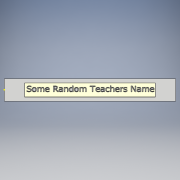
# Autodesk Inventor part: NameTag
Saved by Autodesk Inventor 2018 (Build 220112000, 112)
## iProperties
Created: 2019-03-18
Part Number: NameTag
Material: Generic
Document SubType Name: Modeling
Designer: This kid
Density: 1 g/cm^3
Appearance: Default
Author: This kid
Autodesk Inventor part; units mm, degrees
(part 1 of 2)
ref_plane "YZ Plane" through (0, 0, 0) normal (1, 0, 0) x (0, 1, 0)
ref_plane "XZ Plane" through (0, 0, 0) normal (0, 1, 0) x (-1, 0, 0)
ref_plane "XY Plane" through (0, 0, 0) normal (0, 0, 1) x (1, 0, 0)
sketch "Sketch1" plane through (0, 0, 0) normal (0, 0, 1) x (1, 0, 0)
  line L0 (0, 6.6514) -> (5.7603, -3.3257)
  line L1 (5.7603, -3.3257) -> (-5.7603, -3.3257)
  line L2 (-5.7603, -3.3257) -> (0, 6.6514)
  point P0 (0, 0)
  point P1 (0, 0)
  constraints: 6 end point, 1 coincident, 7 other
extrude "Extrusion1" add sketch "Sketch1" along normal blind 76.2
sketch "Sketch2" plane through (-5.7603, -3.3257, 0) normal (-0.8660254, 0.5, 0) x (0, 0, 1)
  line L0 (9.0292, 2.0917) -> (67.1704, 2.0917)
  line L1 (67.1704, 2.0917) -> (67.1704, 9.2481)
  line L2 (67.1704, 9.2481) -> (9.0292, 9.2481)
  line L3 (9.0292, 9.2481) -> (9.0292, 2.0917)
  line L4 (0, 5.7603) -> (9.0292, 5.6699) construction
  line L5 (67.1704, 5.7603) -> (76.2, 5.7603) construction
  constraints: 12 end point, 2 parallel, 1 equal length, 1 horizontal, 1 midpoint, 1 perpendicular, 1 point on line
extrude "Extrusion2" add sketch "Sketch2" along normal blind 0.2286
sketch "Sketch3" plane through (-5.9582, -3.2114, 0) normal (-0.8660254, 0.5, 0) x (0, 0, 1)
  point P0 (0, 5.7603)
sketch "Sketch4" plane through (-5.9582, -3.2114, 0) normal (-0.8660254, 0.5, 0) x (0, 0, 1)
  line L0 (9.8332, 7.8709) -> (68.5929, 7.8709) construction
  line L1 (68.5929, 7.8709) -> (68.5929, 1.5104) construction
  line L2 (68.5929, 1.5104) -> (9.8332, 1.5104) construction
  line L3 (9.8332, 1.5104) -> (9.8332, 7.8709) construction
  spline S0 degree 2 poles (10.9916, 4.6327) (10.6607, 4.6327) (10.1963, 4.7711) (9.9913, 4.8699) knots 0 0 0 1 2 2 2
  line L4 (9.9913, 4.8699) -> (9.9913, 5.3787)
  line L5 (9.9913, 5.3787) -> (10.0209, 5.3787)
  spline S1 degree 2 poles (10.0209, 5.3787) (10.221, 5.191) (10.7274, 4.9835) (10.962, 4.9835) knots 0 0 0 1 2 2 2
  spline S2 degree 2 poles (10.962, 4.9835) (11.2979, 4.9835) (11.6413, 5.2626) (11.6413, 5.4923) knots 0 0 0 1 2 2 2
  spline S3 degree 2 poles (11.6413, 5.4923) (11.6413, 5.6751) (11.4609, 5.9023) (11.2658, 5.9591) knots 0 0 0 1 2 2 2
  spline S4 degree 2 poles (11.2658, 5.9591) (11.125, 5.9987) (10.8904, 6.053) (10.715, 6.0975) knots 0 0 0 1 2 2 2
  spline S5 degree 2 poles (10.715, 6.0975) (10.5569, 6.1394) (10.3075, 6.2654) (10.2111, 6.3667) knots 0 0 0 1 2 2 2
  spline S6 degree 2 poles (10.2111, 6.3667) (10.1173, 6.468) (10.0135, 6.7397) (10.0135, 6.9175) knots 0 0 0 1 2 2 2
  spline S7 degree 2 poles (10.0135, 6.9175) (10.0135, 7.288) (10.5915, 7.7894) (11.0386, 7.7894) knots 0 0 0 1 2 2 2
  spline S8 degree 2 poles (11.0386, 7.7894) (11.2955, 7.7894) (11.7499, 7.6881) (11.9451, 7.5918) knots 0 0 0 1 2 2 2
  line L6 (11.9451, 7.5918) -> (11.9451, 7.1077)
  line L7 (11.9451, 7.1077) -> (11.9154, 7.1077)
  spline S9 degree 2 poles (11.9154, 7.1077) (11.7697, 7.2411) (11.3152, 7.4387) (11.0657, 7.4387) knots 0 0 0 1 2 2 2
  spline S10 degree 2 poles (11.0657, 7.4387) (10.7842, 7.4387) (10.4359, 7.1744) (10.4359, 6.9595) knots 0 0 0 1 2 2 2
  spline S11 degree 2 poles (10.4359, 6.9595) (10.4359, 6.7668) (10.6409, 6.5371) (10.8336, 6.4852) knots 0 0 0 1 2 2 2
  spline S12 degree 2 poles (10.8336, 6.4852) (10.962, 6.4507) (11.335, 6.3617) (11.4585, 6.3247) knots 0 0 0 1 2 2 2
  spline S13 degree 2 poles (11.4585, 6.3247) (11.7722, 6.2284) (12.0636, 5.8406) (12.0636, 5.5565) knots 0 0 0 1 2 2 2
  spline S14 degree 2 poles (12.0636, 5.5565) (12.0636, 5.3762) (11.9179, 5.0304) (11.787, 4.9094) knots 0 0 0 1 2 2 2
  spline S15 degree 2 poles (11.787, 4.9094) (11.6413, 4.776) (11.2708, 4.6327) (10.9916, 4.6327) knots 0 0 0 1 2 2 2
  spline S16 degree 2 poles (14.3262, 5.8307) (14.3262, 5.2527) (13.7704, 4.6229) (13.3061, 4.6229) knots 0 0 0 1 2 2 2
  spline S17 degree 2 poles (13.3061, 4.6229) (12.8293, 4.6229) (12.2835, 5.2725) (12.2835, 5.8307) knots 0 0 0 1 2 2 2
  spline S18 degree 2 poles (12.2835, 5.8307) (12.2835, 6.4037) (12.8466, 7.0385) (13.3061, 7.0385) knots 0 0 0 1 2 2 2
  spline S19 degree 2 poles (13.3061, 7.0385) (13.7704, 7.0385) (14.3262, 6.4062) (14.3262, 5.8307) knots 0 0 0 1 2 2 2
  spline S20 degree 2 poles (13.9285, 5.8307) (13.9285, 6.2753) (13.6049, 6.7075) (13.3061, 6.7075) knots 0 0 0 1 2 2 2
  spline S21 degree 2 poles (13.3061, 6.7075) (13.0072, 6.7075) (12.6811, 6.2753) (12.6811, 5.8307) knots 0 0 0 1 2 2 2
  spline S22 degree 2 poles (12.6811, 5.8307) (12.6811, 5.3984) (13.0072, 4.9538) (13.3061, 4.9538) knots 0 0 0 1 2 2 2
  spline S23 degree 2 poles (13.3061, 4.9538) (13.6025, 4.9538) (13.9285, 5.391) (13.9285, 5.8307) knots 0 0 0 1 2 2 2
  line L8 (17.3149, 4.6871) -> (17.3149, 6.011)
  spline S24 degree 2 poles (17.3149, 6.011) (17.3149, 6.1691) (17.2902, 6.4383) (17.2507, 6.5124) knots 0 0 0 1 2 2 2
  spline S25 degree 2 poles (17.2507, 6.5124) (17.2111, 6.5939) (17.0605, 6.673) (16.9296, 6.673) knots 0 0 0 1 2 2 2
  spline S26 degree 2 poles (16.9296, 6.673) (16.811, 6.673) (16.5393, 6.5272) (16.396, 6.3889) knots 0 0 0 1 2 2 2
  spline S27 degree 2 poles (16.396, 6.3889) (16.3985, 6.3543) (16.4035, 6.258) (16.4035, 6.1938) knots 0 0 0 1 2 2 2
  line L9 (16.4035, 6.1938) -> (16.4035, 4.6871)
  line L10 (16.4035, 4.6871) -> (16.0181, 4.6871)
  line L11 (16.0181, 4.6871) -> (16.0181, 6.011)
  spline S28 degree 2 poles (16.0181, 6.011) (16.0181, 6.1691) (15.9934, 6.4383) (15.9539, 6.5124) knots 0 0 0 1 2 2 2
  spline S29 degree 2 poles (15.9539, 6.5124) (15.9144, 6.5939) (15.7637, 6.673) (15.6328, 6.673) knots 0 0 0 1 2 2 2
  spline S30 degree 2 poles (15.6328, 6.673) (15.5093, 6.673) (15.2351, 6.5174) (15.1067, 6.3963) knots 0 0 0 1 2 2 2
  line L12 (15.1067, 6.3963) -> (15.1067, 4.6871)
  line L13 (15.1067, 4.6871) -> (14.7214, 4.6871)
  line L14 (14.7214, 4.6871) -> (14.7214, 6.9743)
  line L15 (14.7214, 6.9743) -> (15.1067, 6.9743)
  line L16 (15.1067, 6.9743) -> (15.1067, 6.7224)
  spline S31 degree 2 poles (15.1067, 6.7224) (15.2574, 6.873) (15.5538, 7.0385) (15.7316, 7.0385) knots 0 0 0 1 2 2 2
  spline S32 degree 2 poles (15.7316, 7.0385) (15.9341, 7.0385) (16.2478, 6.8533) (16.3294, 6.6433) knots 0 0 0 1 2 2 2
  spline S33 degree 2 poles (16.3294, 6.6433) (16.5047, 6.8385) (16.8357, 7.0385) (17.0284, 7.0385) knots 0 0 0 1 2 2 2
  spline S34 degree 2 poles (17.0284, 7.0385) (17.1766, 7.0385) (17.4186, 6.9471) (17.5075, 6.8434) knots 0 0 0 1 2 2 2
  spline S35 degree 2 poles (17.5075, 6.8434) (17.5989, 6.7397) (17.7002, 6.4284) (17.7002, 6.1938) knots 0 0 0 1 2 2 2
  line L17 (17.7002, 6.1938) -> (17.7002, 4.6871)
  line L18 (17.7002, 4.6871) -> (17.3149, 4.6871)
  spline S36 degree 2 poles (19.2341, 4.6352) (18.6857, 4.6352) (18.0831, 5.2502) (18.0831, 5.8183) knots 0 0 0 1 2 2 2
  spline S37 degree 2 poles (18.0831, 5.8183) (18.0831, 6.3766) (18.6685, 7.0385) (19.1402, 7.0385) knots 0 0 0 1 2 2 2
  spline S38 degree 2 poles (19.1402, 7.0385) (19.3527, 7.0385) (19.6812, 6.915) (19.8022, 6.7841) knots 0 0 0 1 2 2 2
  spline S39 degree 2 poles (19.8022, 6.7841) (19.9257, 6.6532) (20.0566, 6.2753) (20.0566, 6.0011) knots 0 0 0 1 2 2 2
  line L19 (20.0566, 6.0011) -> (20.0566, 5.7912)
  line L20 (20.0566, 5.7912) -> (18.4733, 5.7912)
  spline S40 degree 2 poles (18.4733, 5.7912) (18.4733, 5.3935) (18.8735, 4.9711) (19.2292, 4.9711) knots 0 0 0 1 2 2 2
  spline S41 degree 2 poles (19.2292, 4.9711) (19.3551, 4.9711) (19.5997, 5.0279) (19.6985, 5.0724) knots 0 0 0 1 2 2 2
  spline S42 degree 2 poles (19.6985, 5.0724) (19.8022, 5.1218) (19.9455, 5.2082) (19.9924, 5.2478) knots 0 0 0 1 2 2 2
  line L21 (19.9924, 5.2478) -> (20.0146, 5.2478)
  line L22 (20.0146, 5.2478) -> (20.0146, 4.8279)
  spline S43 degree 2 poles (20.0146, 4.8279) (19.9479, 4.8007) (19.7454, 4.7217) (19.6663, 4.6994) knots 0 0 0 1 2 2 2
  spline S44 degree 2 poles (19.6663, 4.6994) (19.5552, 4.6673) (19.3724, 4.6352) (19.2341, 4.6352) knots 0 0 0 1 2 2 2
  spline S45 degree 2 poles (19.6812, 6.0851) (19.6762, 6.2407) (19.612, 6.468) (19.5503, 6.5445) knots 0 0 0 1 2 2 2
  spline S46 degree 2 poles (19.5503, 6.5445) (19.4836, 6.631) (19.2736, 6.7224) (19.118, 6.7224) knots 0 0 0 1 2 2 2
  spline S47 degree 2 poles (19.118, 6.7224) (18.9649, 6.7224) (18.75, 6.631) (18.661, 6.5421) knots 0 0 0 1 2 2 2
  spline S48 degree 2 poles (18.661, 6.5421) (18.5746, 6.4507) (18.4857, 6.2308) (18.4733, 6.0851) knots 0 0 0 1 2 2 2
  line L23 (18.4733, 6.0851) -> (19.6812, 6.0851)
  line L24 (24.1445, 4.6871) -> (23.6184, 4.6871)
  line L25 (23.6184, 4.6871) -> (22.6551, 5.8999)
  line L26 (22.6551, 5.8999) -> (22.1907, 5.8999)
  line L27 (22.1907, 5.8999) -> (22.1907, 4.6871)
  line L28 (22.1907, 4.6871) -> (21.7856, 4.6871)
  line L29 (21.7856, 4.6871) -> (21.7856, 7.7351)
  line L30 (21.7856, 7.7351) -> (22.5711, 7.7351)
  spline S49 degree 2 poles (22.5711, 7.7351) (22.8329, 7.7351) (23.1861, 7.6783) (23.3467, 7.5745) knots 0 0 0 1 2 2 2
  spline S50 degree 2 poles (23.3467, 7.5745) (23.5072, 7.4708) (23.6925, 7.1472) (23.6925, 6.9076) knots 0 0 0 1 2 2 2
  spline S51 degree 2 poles (23.6925, 6.9076) (23.6925, 6.5742) (23.3516, 6.1222) (23.0601, 6.0135) knots 0 0 0 1 2 2 2
  line L31 (23.0601, 6.0135) -> (24.1445, 4.6871)
  spline S52 degree 2 poles (23.2701, 6.8755) (23.2701, 7.0089) (23.1762, 7.2139) (23.0774, 7.2806) knots 0 0 0 1 2 2 2
  spline S53 degree 2 poles (23.0774, 7.2806) (22.991, 7.3374) (22.7613, 7.3843) (22.5933, 7.3843) knots 0 0 0 1 2 2 2
  line L32 (22.5933, 7.3843) -> (22.1907, 7.3843)
  line L33 (22.1907, 7.3843) -> (22.1907, 6.2382)
  line L34 (22.1907, 6.2382) -> (22.5464, 6.2382)
  spline S54 degree 2 poles (22.5464, 6.2382) (22.7218, 6.2382) (23.0009, 6.3) (23.0972, 6.3963) knots 0 0 0 1 2 2 2
  spline S55 degree 2 poles (23.0972, 6.3963) (23.1861, 6.4803) (23.2701, 6.7174) (23.2701, 6.8755) knots 0 0 0 1 2 2 2
  spline S56 degree 2 poles (25.6314, 4.9291) (25.5845, 4.8946) (25.4264, 4.7711) (25.3523, 4.734) knots 0 0 0 1 2 2 2
  spline S57 degree 2 poles (25.3523, 4.734) (25.2511, 4.6797) (25.0609, 4.6229) (24.888, 4.6229) knots 0 0 0 1 2 2 2
  spline S58 degree 2 poles (24.888, 4.6229) (24.7472, 4.6229) (24.4928, 4.7291) (24.3964, 4.8254) knots 0 0 0 1 2 2 2
  spline S59 degree 2 poles (24.3964, 4.8254) (24.305, 4.9193) (24.1939, 5.1959) (24.1939, 5.349) knots 0 0 0 1 2 2 2
  spline S60 degree 2 poles (24.1939, 5.349) (24.1939, 5.5862) (24.394, 5.9221) (24.6113, 6.0184) knots 0 0 0 1 2 2 2
  spline S61 degree 2 poles (24.6113, 6.0184) (24.804, 6.1073) (25.3276, 6.174) (25.6314, 6.1913) knots 0 0 0 1 2 2 2
  line L35 (25.6314, 6.1913) -> (25.6314, 6.2654)
  spline S62 degree 2 poles (25.6314, 6.2654) (25.6314, 6.3988) (25.5499, 6.5643) (25.4758, 6.6112) knots 0 0 0 1 2 2 2
  spline S63 degree 2 poles (25.4758, 6.6112) (25.4017, 6.6581) (25.1893, 6.6878) (25.0757, 6.6878) knots 0 0 0 1 2 2 2
  spline S64 degree 2 poles (25.0757, 6.6878) (24.9423, 6.6878) (24.5817, 6.6087) (24.4014, 6.5322) knots 0 0 0 1 2 2 2
  line L36 (24.4014, 6.5322) -> (24.3791, 6.5322)
  line L37 (24.3791, 6.5322) -> (24.3791, 6.9249)
  spline S65 degree 2 poles (24.3791, 6.9249) (24.4853, 6.9546) (24.883, 7.0287) (25.0781, 7.0287) knots 0 0 0 1 2 2 2
  spline S66 degree 2 poles (25.0781, 7.0287) (25.3153, 7.0287) (25.6388, 6.9546) (25.7673, 6.8582) knots 0 0 0 1 2 2 2
  spline S67 degree 2 poles (25.7673, 6.8582) (25.8933, 6.7644) (26.0168, 6.4655) (26.0168, 6.2506) knots 0 0 0 1 2 2 2
  line L38 (26.0168, 6.2506) -> (26.0168, 4.6871)
  line L39 (26.0168, 4.6871) -> (25.6314, 4.6871)
  line L40 (25.6314, 4.6871) -> (25.6314, 4.9291)
  line L41 (25.6314, 5.2502) -> (25.6314, 5.885)
  spline S68 degree 2 poles (25.6314, 5.885) (25.4931, 5.8727) (25.0757, 5.8307) (24.9448, 5.7912) knots 0 0 0 1 2 2 2
  spline S69 degree 2 poles (24.9448, 5.7912) (24.7916, 5.7442) (24.5916, 5.5491) (24.5916, 5.3762) knots 0 0 0 1 2 2 2
  spline S70 degree 2 poles (24.5916, 5.3762) (24.5916, 5.1786) (24.8139, 4.9785) (25.0263, 4.9785) knots 0 0 0 1 2 2 2
  spline S71 degree 2 poles (25.0263, 4.9785) (25.2066, 4.9785) (25.503, 5.1341) (25.6314, 5.2502) knots 0 0 0 1 2 2 2
  line L42 (28.3534, 4.6871) -> (27.9681, 4.6871)
  line L43 (27.9681, 4.6871) -> (27.9681, 5.9912)
  spline S72 degree 2 poles (27.9681, 5.9912) (27.9681, 6.1493) (27.9384, 6.421) (27.894, 6.5025) knots 0 0 0 1 2 2 2
  spline S73 degree 2 poles (27.894, 6.5025) (27.847, 6.589) (27.6791, 6.673) (27.5358, 6.673) knots 0 0 0 1 2 2 2
  spline S74 degree 2 poles (27.5358, 6.673) (27.3926, 6.673) (27.0887, 6.5198) (26.943, 6.3963) knots 0 0 0 1 2 2 2
  line L44 (26.943, 6.3963) -> (26.943, 4.6871)
  line L45 (26.943, 4.6871) -> (26.5577, 4.6871)
  line L46 (26.5577, 4.6871) -> (26.5577, 6.9743)
  line L47 (26.5577, 6.9743) -> (26.943, 6.9743)
  line L48 (26.943, 6.9743) -> (26.943, 6.7199)
  spline S75 degree 2 poles (26.943, 6.7199) (27.1159, 6.8755) (27.4494, 7.0385) (27.6371, 7.0385) knots 0 0 0 1 2 2 2
  spline S76 degree 2 poles (27.6371, 7.0385) (27.973, 7.0385) (28.3534, 6.5939) (28.3534, 6.1716) knots 0 0 0 1 2 2 2
  line L49 (28.3534, 6.1716) -> (28.3534, 4.6871)
  line L50 (30.653, 4.6871) -> (30.2677, 4.6871)
  line L51 (30.2677, 4.6871) -> (30.2677, 4.9193)
  spline S77 degree 2 poles (30.2677, 4.9193) (30.1787, 4.8452) (30.0478, 4.7464) (29.9589, 4.7044) knots 0 0 0 1 2 2 2
  spline S78 degree 2 poles (29.9589, 4.7044) (29.8774, 4.6648) (29.702, 4.6229) (29.5859, 4.6229) knots 0 0 0 1 2 2 2
  spline S79 degree 2 poles (29.5859, 4.6229) (29.3982, 4.6229) (29.082, 4.7785) (28.9709, 4.9291) knots 0 0 0 1 2 2 2
  spline S80 degree 2 poles (28.9709, 4.9291) (28.8597, 5.0798) (28.7362, 5.5244) (28.7362, 5.8134) knots 0 0 0 1 2 2 2
  spline S81 degree 2 poles (28.7362, 5.8134) (28.7362, 6.1147) (28.8919, 6.5544) (29.0277, 6.7199) knots 0 0 0 1 2 2 2
  spline S82 degree 2 poles (29.0277, 6.7199) (29.1537, 6.8681) (29.5069, 7.0385) (29.702, 7.0385) knots 0 0 0 1 2 2 2
  spline S83 degree 2 poles (29.702, 7.0385) (29.8725, 7.0385) (30.1269, 6.962) (30.2677, 6.8829) knots 0 0 0 1 2 2 2
  line L52 (30.2677, 6.8829) -> (30.2677, 7.8709)
  line L53 (30.2677, 7.8709) -> (30.653, 7.8709)
  line L54 (30.653, 7.8709) -> (30.653, 4.6871)
  line L55 (30.2677, 5.2428) -> (30.2677, 6.5643)
  spline S84 degree 2 poles (30.2677, 6.5643) (30.1244, 6.6334) (29.8972, 6.6853) (29.7662, 6.6853) knots 0 0 0 1 2 2 2
  spline S85 degree 2 poles (29.7662, 6.6853) (29.4698, 6.6853) (29.1339, 6.2407) (29.1339, 5.8208) knots 0 0 0 1 2 2 2
  spline S86 degree 2 poles (29.1339, 5.8208) (29.1339, 5.4157) (29.3908, 4.9884) (29.6748, 4.9884) knots 0 0 0 1 2 2 2
  spline S87 degree 2 poles (29.6748, 4.9884) (29.8255, 4.9884) (30.1318, 5.1267) (30.2677, 5.2428) knots 0 0 0 1 2 2 2
  spline S88 degree 2 poles (33.0909, 5.8307) (33.0909, 5.2527) (32.5351, 4.6229) (32.0708, 4.6229) knots 0 0 0 1 2 2 2
  spline S89 degree 2 poles (32.0708, 4.6229) (31.5941, 4.6229) (31.0482, 5.2725) (31.0482, 5.8307) knots 0 0 0 1 2 2 2
  spline S90 degree 2 poles (31.0482, 5.8307) (31.0482, 6.4037) (31.6113, 7.0385) (32.0708, 7.0385) knots 0 0 0 1 2 2 2
  spline S91 degree 2 poles (32.0708, 7.0385) (32.5351, 7.0385) (33.0909, 6.4062) (33.0909, 5.8307) knots 0 0 0 1 2 2 2
  spline S92 degree 2 poles (32.6932, 5.8307) (32.6932, 6.2753) (32.3696, 6.7075) (32.0708, 6.7075) knots 0 0 0 1 2 2 2
  spline S93 degree 2 poles (32.0708, 6.7075) (31.7719, 6.7075) (31.4459, 6.2753) (31.4459, 5.8307) knots 0 0 0 1 2 2 2
  spline S94 degree 2 poles (31.4459, 5.8307) (31.4459, 5.3984) (31.7719, 4.9538) (32.0708, 4.9538) knots 0 0 0 1 2 2 2
  spline S95 degree 2 poles (32.0708, 4.9538) (32.3672, 4.9538) (32.6932, 5.391) (32.6932, 5.8307) knots 0 0 0 1 2 2 2
  line L56 (36.0796, 4.6871) -> (36.0796, 6.011)
  spline S96 degree 2 poles (36.0796, 6.011) (36.0796, 6.1691) (36.0549, 6.4383) (36.0154, 6.5124) knots 0 0 0 1 2 2 2
  spline S97 degree 2 poles (36.0154, 6.5124) (35.9759, 6.5939) (35.8252, 6.673) (35.6943, 6.673) knots 0 0 0 1 2 2 2
  spline S98 degree 2 poles (35.6943, 6.673) (35.5757, 6.673) (35.304, 6.5272) (35.1608, 6.3889) knots 0 0 0 1 2 2 2
  spline S99 degree 2 poles (35.1608, 6.3889) (35.1632, 6.3543) (35.1682, 6.258) (35.1682, 6.1938) knots 0 0 0 1 2 2 2
  line L57 (35.1682, 6.1938) -> (35.1682, 4.6871)
  line L58 (35.1682, 4.6871) -> (34.7828, 4.6871)
  line L59 (34.7828, 4.6871) -> (34.7828, 6.011)
  spline S100 degree 2 poles (34.7828, 6.011) (34.7828, 6.1691) (34.7581, 6.4383) (34.7186, 6.5124) knots 0 0 0 1 2 2 2
  spline S101 degree 2 poles (34.7186, 6.5124) (34.6791, 6.5939) (34.5284, 6.673) (34.3975, 6.673) knots 0 0 0 1 2 2 2
  spline S102 degree 2 poles (34.3975, 6.673) (34.274, 6.673) (33.9998, 6.5174) (33.8714, 6.3963) knots 0 0 0 1 2 2 2
  line L60 (33.8714, 6.3963) -> (33.8714, 4.6871)
  line L61 (33.8714, 4.6871) -> (33.4861, 4.6871)
  line L62 (33.4861, 4.6871) -> (33.4861, 6.9743)
  line L63 (33.4861, 6.9743) -> (33.8714, 6.9743)
  line L64 (33.8714, 6.9743) -> (33.8714, 6.7224)
  spline S103 degree 2 poles (33.8714, 6.7224) (34.0221, 6.873) (34.3185, 7.0385) (34.4963, 7.0385) knots 0 0 0 1 2 2 2
  spline S104 degree 2 poles (34.4963, 7.0385) (34.6989, 7.0385) (35.0126, 6.8533) (35.0941, 6.6433) knots 0 0 0 1 2 2 2
  spline S105 degree 2 poles (35.0941, 6.6433) (35.2694, 6.8385) (35.6004, 7.0385) (35.7931, 7.0385) knots 0 0 0 1 2 2 2
  spline S106 degree 2 poles (35.7931, 7.0385) (35.9413, 7.0385) (36.1833, 6.9471) (36.2723, 6.8434) knots 0 0 0 1 2 2 2
  spline S107 degree 2 poles (36.2723, 6.8434) (36.3637, 6.7397) (36.4649, 6.4284) (36.4649, 6.1938) knots 0 0 0 1 2 2 2
  line L65 (36.4649, 6.1938) -> (36.4649, 4.6871)
  line L66 (36.4649, 4.6871) -> (36.0796, 4.6871)
  line L67 (39.056, 4.6871) -> (39.056, 7.3745)
  line L68 (39.056, 7.3745) -> (38.0334, 7.3745)
  line L69 (38.0334, 7.3745) -> (38.0334, 7.7351)
  line L70 (38.0334, 7.7351) -> (40.4836, 7.7351)
  line L71 (40.4836, 7.7351) -> (40.4836, 7.3745)
  line L72 (40.4836, 7.3745) -> (39.4611, 7.3745)
  line L73 (39.4611, 7.3745) -> (39.4611, 4.6871)
  line L74 (39.4611, 4.6871) -> (39.056, 4.6871)
  spline S108 degree 2 poles (41.7557, 4.6352) (41.2074, 4.6352) (40.6047, 5.2502) (40.6047, 5.8183) knots 0 0 0 1 2 2 2
  spline S109 degree 2 poles (40.6047, 5.8183) (40.6047, 6.3766) (41.1901, 7.0385) (41.6618, 7.0385) knots 0 0 0 1 2 2 2
  spline S110 degree 2 poles (41.6618, 7.0385) (41.8743, 7.0385) (42.2028, 6.915) (42.3238, 6.7841) knots 0 0 0 1 2 2 2
  spline S111 degree 2 poles (42.3238, 6.7841) (42.4473, 6.6532) (42.5782, 6.2753) (42.5782, 6.0011) knots 0 0 0 1 2 2 2
  line L75 (42.5782, 6.0011) -> (42.5782, 5.7912)
  line L76 (42.5782, 5.7912) -> (40.9949, 5.7912)
  spline S112 degree 2 poles (40.9949, 5.7912) (40.9949, 5.3935) (41.3951, 4.9711) (41.7508, 4.9711) knots 0 0 0 1 2 2 2
  spline S113 degree 2 poles (41.7508, 4.9711) (41.8767, 4.9711) (42.1213, 5.0279) (42.2201, 5.0724) knots 0 0 0 1 2 2 2
  spline S114 degree 2 poles (42.2201, 5.0724) (42.3238, 5.1218) (42.4671, 5.2082) (42.514, 5.2478) knots 0 0 0 1 2 2 2
  line L77 (42.514, 5.2478) -> (42.5362, 5.2478)
  line L78 (42.5362, 5.2478) -> (42.5362, 4.8279)
  spline S115 degree 2 poles (42.5362, 4.8279) (42.4695, 4.8007) (42.267, 4.7217) (42.188, 4.6994) knots 0 0 0 1 2 2 2
  spline S116 degree 2 poles (42.188, 4.6994) (42.0768, 4.6673) (41.894, 4.6352) (41.7557, 4.6352) knots 0 0 0 1 2 2 2
  spline S117 degree 2 poles (42.2028, 6.0851) (42.1978, 6.2407) (42.1336, 6.468) (42.0719, 6.5445) knots 0 0 0 1 2 2 2
  spline S118 degree 2 poles (42.0719, 6.5445) (42.0052, 6.631) (41.7952, 6.7224) (41.6396, 6.7224) knots 0 0 0 1 2 2 2
  spline S119 degree 2 poles (41.6396, 6.7224) (41.4865, 6.7224) (41.2716, 6.631) (41.1827, 6.5421) knots 0 0 0 1 2 2 2
  spline S120 degree 2 poles (41.1827, 6.5421) (41.0962, 6.4507) (41.0073, 6.2308) (40.9949, 6.0851) knots 0 0 0 1 2 2 2
  line L79 (40.9949, 6.0851) -> (42.2028, 6.0851)
  spline S121 degree 2 poles (44.243, 4.9291) (44.1961, 4.8946) (44.038, 4.7711) (43.9639, 4.734) knots 0 0 0 1 2 2 2
  spline S122 degree 2 poles (43.9639, 4.734) (43.8626, 4.6797) (43.6724, 4.6229) (43.4995, 4.6229) knots 0 0 0 1 2 2 2
  spline S123 degree 2 poles (43.4995, 4.6229) (43.3587, 4.6229) (43.1043, 4.7291) (43.008, 4.8254) knots 0 0 0 1 2 2 2
  spline S124 degree 2 poles (43.008, 4.8254) (42.9166, 4.9193) (42.8055, 5.1959) (42.8055, 5.349) knots 0 0 0 1 2 2 2
  spline S125 degree 2 poles (42.8055, 5.349) (42.8055, 5.5862) (43.0055, 5.9221) (43.2229, 6.0184) knots 0 0 0 1 2 2 2
  spline S126 degree 2 poles (43.2229, 6.0184) (43.4156, 6.1073) (43.9392, 6.174) (44.243, 6.1913) knots 0 0 0 1 2 2 2
  line L80 (44.243, 6.1913) -> (44.243, 6.2654)
  spline S127 degree 2 poles (44.243, 6.2654) (44.243, 6.3988) (44.1615, 6.5643) (44.0874, 6.6112) knots 0 0 0 1 2 2 2
  spline S128 degree 2 poles (44.0874, 6.6112) (44.0133, 6.6581) (43.8009, 6.6878) (43.6873, 6.6878) knots 0 0 0 1 2 2 2
  spline S129 degree 2 poles (43.6873, 6.6878) (43.5539, 6.6878) (43.1932, 6.6087) (43.0129, 6.5322) knots 0 0 0 1 2 2 2
  line L81 (43.0129, 6.5322) -> (42.9907, 6.5322)
  line L82 (42.9907, 6.5322) -> (42.9907, 6.9249)
  spline S130 degree 2 poles (42.9907, 6.9249) (43.0969, 6.9546) (43.4946, 7.0287) (43.6897, 7.0287) knots 0 0 0 1 2 2 2
  spline S131 degree 2 poles (43.6897, 7.0287) (43.9268, 7.0287) (44.2504, 6.9546) (44.3789, 6.8582) knots 0 0 0 1 2 2 2
  spline S132 degree 2 poles (44.3789, 6.8582) (44.5048, 6.7644) (44.6283, 6.4655) (44.6283, 6.2506) knots 0 0 0 1 2 2 2
  line L83 (44.6283, 6.2506) -> (44.6283, 4.6871)
  line L84 (44.6283, 4.6871) -> (44.243, 4.6871)
  line L85 (44.243, 4.6871) -> (44.243, 4.9291)
  line L86 (44.243, 5.2502) -> (44.243, 5.885)
  spline S133 degree 2 poles (44.243, 5.885) (44.1047, 5.8727) (43.6873, 5.8307) (43.5563, 5.7912) knots 0 0 0 1 2 2 2
  spline S134 degree 2 poles (43.5563, 5.7912) (43.4032, 5.7442) (43.2031, 5.5491) (43.2031, 5.3762) knots 0 0 0 1 2 2 2
  spline S135 degree 2 poles (43.2031, 5.3762) (43.2031, 5.1786) (43.4254, 4.9785) (43.6379, 4.9785) knots 0 0 0 1 2 2 2
  spline S136 degree 2 poles (43.6379, 4.9785) (43.8182, 4.9785) (44.1146, 5.1341) (44.243, 5.2502) knots 0 0 0 1 2 2 2
  spline S137 degree 2 poles (46.0782, 4.6352) (45.8411, 4.6352) (45.4484, 4.7809) (45.3076, 4.9291) knots 0 0 0 1 2 2 2
  spline S138 degree 2 poles (45.3076, 4.9291) (45.1668, 5.0749) (45.0112, 5.5244) (45.0112, 5.8258) knots 0 0 0 1 2 2 2
  spline S139 degree 2 poles (45.0112, 5.8258) (45.0112, 6.1271) (45.1717, 6.5668) (45.3076, 6.715) knots 0 0 0 1 2 2 2
  spline S140 degree 2 poles (45.3076, 6.715) (45.4434, 6.8656) (45.846, 7.0262) (46.0782, 7.0262) knots 0 0 0 1 2 2 2
  spline S141 degree 2 poles (46.0782, 7.0262) (46.2659, 7.0262) (46.6167, 6.92) (46.7525, 6.8508) knots 0 0 0 1 2 2 2
  line L87 (46.7525, 6.8508) -> (46.7525, 6.4186)
  line L88 (46.7525, 6.4186) -> (46.7303, 6.4186)
  spline S142 degree 2 poles (46.7303, 6.4186) (46.6883, 6.4531) (46.5599, 6.5421) (46.4685, 6.589) knots 0 0 0 1 2 2 2
  spline S143 degree 2 poles (46.4685, 6.589) (46.387, 6.6285) (46.1696, 6.6903) (46.0708, 6.6903) knots 0 0 0 1 2 2 2
  spline S144 degree 2 poles (46.0708, 6.6903) (45.7719, 6.6903) (45.4089, 6.2382) (45.4089, 5.8258) knots 0 0 0 1 2 2 2
  spline S145 degree 2 poles (45.4089, 5.8258) (45.4089, 5.4231) (45.7596, 4.9711) (46.0708, 4.9711) knots 0 0 0 1 2 2 2
  spline S146 degree 2 poles (46.0708, 4.9711) (46.2585, 4.9711) (46.5994, 5.1267) (46.7303, 5.2478) knots 0 0 0 1 2 2 2
  line L89 (46.7303, 5.2478) -> (46.7525, 5.2478)
  line L90 (46.7525, 5.2478) -> (46.7525, 4.8155)
  spline S147 degree 2 poles (46.7525, 4.8155) (46.6957, 4.7883) (46.5228, 4.7118) (46.4537, 4.6945) knots 0 0 0 1 2 2 2
  spline S148 degree 2 poles (46.4537, 4.6945) (46.3549, 4.6648) (46.1993, 4.6352) (46.0782, 4.6352) knots 0 0 0 1 2 2 2
  line L91 (48.899, 4.6871) -> (48.5137, 4.6871)
  line L92 (48.5137, 4.6871) -> (48.5137, 5.9912)
  spline S149 degree 2 poles (48.5137, 5.9912) (48.5137, 6.1493) (48.484, 6.421) (48.4396, 6.5025) knots 0 0 0 1 2 2 2
  spline S150 degree 2 poles (48.4396, 6.5025) (48.3926, 6.589) (48.2247, 6.673) (48.0814, 6.673) knots 0 0 0 1 2 2 2
  spline S151 degree 2 poles (48.0814, 6.673) (47.9381, 6.673) (47.6343, 6.5198) (47.4886, 6.3963) knots 0 0 0 1 2 2 2
  line L93 (47.4886, 6.3963) -> (47.4886, 4.6871)
  line L94 (47.4886, 4.6871) -> (47.1033, 4.6871)
  line L95 (47.1033, 4.6871) -> (47.1033, 7.8709)
  line L96 (47.1033, 7.8709) -> (47.4886, 7.8709)
  line L97 (47.4886, 7.8709) -> (47.4886, 6.7199)
  spline S152 degree 2 poles (47.4886, 6.7199) (47.6615, 6.8755) (47.995, 7.0385) (48.1827, 7.0385) knots 0 0 0 1 2 2 2
  spline S153 degree 2 poles (48.1827, 7.0385) (48.5186, 7.0385) (48.899, 6.5939) (48.899, 6.1716) knots 0 0 0 1 2 2 2
  line L98 (48.899, 6.1716) -> (48.899, 4.6871)
  spline S154 degree 2 poles (50.4329, 4.6352) (49.8845, 4.6352) (49.2818, 5.2502) (49.2818, 5.8183) knots 0 0 0 1 2 2 2
  spline S155 degree 2 poles (49.2818, 5.8183) (49.2818, 6.3766) (49.8672, 7.0385) (50.339, 7.0385) knots 0 0 0 1 2 2 2
  spline S156 degree 2 poles (50.339, 7.0385) (50.5514, 7.0385) (50.8799, 6.915) (51.001, 6.7841) knots 0 0 0 1 2 2 2
  spline S157 degree 2 poles (51.001, 6.7841) (51.1245, 6.6532) (51.2554, 6.2753) (51.2554, 6.0011) knots 0 0 0 1 2 2 2
  line L99 (51.2554, 6.0011) -> (51.2554, 5.7912)
  line L100 (51.2554, 5.7912) -> (49.6721, 5.7912)
  spline S158 degree 2 poles (49.6721, 5.7912) (49.6721, 5.3935) (50.0722, 4.9711) (50.4279, 4.9711) knots 0 0 0 1 2 2 2
  spline S159 degree 2 poles (50.4279, 4.9711) (50.5539, 4.9711) (50.7984, 5.0279) (50.8972, 5.0724) knots 0 0 0 1 2 2 2
  spline S160 degree 2 poles (50.8972, 5.0724) (51.001, 5.1218) (51.1442, 5.2082) (51.1912, 5.2478) knots 0 0 0 1 2 2 2
  line L101 (51.1912, 5.2478) -> (51.2134, 5.2478)
  line L102 (51.2134, 5.2478) -> (51.2134, 4.8279)
  spline S161 degree 2 poles (51.2134, 4.8279) (51.1467, 4.8007) (50.9442, 4.7217) (50.8651, 4.6994) knots 0 0 0 1 2 2 2
  spline S162 degree 2 poles (50.8651, 4.6994) (50.754, 4.6673) (50.5712, 4.6352) (50.4329, 4.6352) knots 0 0 0 1 2 2 2
  spline S163 degree 2 poles (50.8799, 6.0851) (50.875, 6.2407) (50.8108, 6.468) (50.749, 6.5445) knots 0 0 0 1 2 2 2
  spline S164 degree 2 poles (50.749, 6.5445) (50.6823, 6.631) (50.4724, 6.7224) (50.3168, 6.7224) knots 0 0 0 1 2 2 2
  spline S165 degree 2 poles (50.3168, 6.7224) (50.1636, 6.7224) (49.9487, 6.631) (49.8598, 6.5421) knots 0 0 0 1 2 2 2
  spline S166 degree 2 poles (49.8598, 6.5421) (49.7734, 6.4507) (49.6845, 6.2308) (49.6721, 6.0851) knots 0 0 0 1 2 2 2
  line L103 (49.6721, 6.0851) -> (50.8799, 6.0851)
  line L104 (52.8584, 6.5618) -> (52.8387, 6.5618)
  spline S167 degree 2 poles (52.8387, 6.5618) (52.7942, 6.5742) (52.6979, 6.5791) (52.6312, 6.5791) knots 0 0 0 1 2 2 2
  spline S168 degree 2 poles (52.6312, 6.5791) (52.4756, 6.5791) (52.1693, 6.4433) (52.031, 6.3099) knots 0 0 0 1 2 2 2
  line L105 (52.031, 6.3099) -> (52.031, 4.6871)
  line L106 (52.031, 4.6871) -> (51.6456, 4.6871)
  line L107 (51.6456, 4.6871) -> (51.6456, 6.9743)
  line L108 (51.6456, 6.9743) -> (52.031, 6.9743)
  line L109 (52.031, 6.9743) -> (52.031, 6.6334)
  spline S169 degree 2 poles (52.031, 6.6334) (52.2409, 6.8212) (52.5546, 6.9743) (52.7028, 6.9743) knots 0 0 0 1 2 2 2
  spline S170 degree 2 poles (52.7028, 6.9743) (52.7621, 6.9743) (52.8214, 6.9694) (52.8584, 6.962) knots 0 0 0 1 2 2 2
  line L110 (52.8584, 6.962) -> (52.8584, 6.5618)
  spline S171 degree 2 poles (53.7748, 4.6327) (53.5451, 4.6327) (53.1474, 4.7562) (53.0165, 4.8254) knots 0 0 0 1 2 2 2
  line L111 (53.0165, 4.8254) -> (53.0165, 5.2577)
  line L112 (53.0165, 5.2577) -> (53.0363, 5.2577)
  spline S172 degree 2 poles (53.0363, 5.2577) (53.0857, 5.2181) (53.219, 5.1243) (53.3302, 5.0724) knots 0 0 0 1 2 2 2
  spline S173 degree 2 poles (53.3302, 5.0724) (53.4265, 5.0255) (53.6636, 4.9563) (53.7896, 4.9563) knots 0 0 0 1 2 2 2
  spline S174 degree 2 poles (53.7896, 4.9563) (53.881, 4.9563) (54.091, 4.9983) (54.1404, 5.0329) knots 0 0 0 1 2 2 2
  spline S175 degree 2 poles (54.1404, 5.0329) (54.212, 5.0798) (54.2762, 5.186) (54.2762, 5.2947) knots 0 0 0 1 2 2 2
  spline S176 degree 2 poles (54.2762, 5.2947) (54.2762, 5.4306) (54.128, 5.5713) (53.9378, 5.6183) knots 0 0 0 1 2 2 2
  spline S177 degree 2 poles (53.9378, 5.6183) (53.8637, 5.6356) (53.6266, 5.685) (53.5253, 5.7121) knots 0 0 0 1 2 2 2
  spline S178 degree 2 poles (53.5253, 5.7121) (53.2635, 5.7887) (53.0264, 6.1049) (53.0264, 6.3296) knots 0 0 0 1 2 2 2
  spline S179 degree 2 poles (53.0264, 6.3296) (53.0264, 6.6409) (53.4932, 7.0287) (53.8785, 7.0287) knots 0 0 0 1 2 2 2
  spline S180 degree 2 poles (53.8785, 7.0287) (54.0687, 7.0287) (54.4541, 6.9348) (54.585, 6.8632) knots 0 0 0 1 2 2 2
  line L113 (54.585, 6.8632) -> (54.585, 6.4507)
  line L114 (54.585, 6.4507) -> (54.5652, 6.4507)
  spline S181 degree 2 poles (54.5652, 6.4507) (54.417, 6.5692) (54.0564, 6.7051) (53.8711, 6.7051) knots 0 0 0 1 2 2 2
  spline S182 degree 2 poles (53.8711, 6.7051) (53.6809, 6.7051) (53.4191, 6.5445) (53.4191, 6.384) knots 0 0 0 1 2 2 2
  spline S183 degree 2 poles (53.4191, 6.384) (53.4191, 6.2382) (53.5747, 6.0975) (53.7476, 6.053) knots 0 0 0 1 2 2 2
  spline S184 degree 2 poles (53.7476, 6.053) (53.8316, 6.0308) (54.044, 5.9863) (54.1601, 5.9591) knots 0 0 0 1 2 2 2
  spline S185 degree 2 poles (54.1601, 5.9591) (54.4121, 5.8949) (54.6689, 5.601) (54.6689, 5.3466) knots 0 0 0 1 2 2 2
  spline S186 degree 2 poles (54.6689, 5.3466) (54.6689, 5.1984) (54.5529, 4.9365) (54.4392, 4.8402) knots 0 0 0 1 2 2 2
  spline S187 degree 2 poles (54.4392, 4.8402) (54.3182, 4.7389) (54.0094, 4.6327) (53.7748, 4.6327) knots 0 0 0 1 2 2 2
  line L115 (58.5469, 4.6871) -> (58.0924, 4.6871)
  line L116 (58.0924, 4.6871) -> (56.7438, 7.3152)
  line L117 (56.7438, 7.3152) -> (56.7438, 4.6871)
  line L118 (56.7438, 4.6871) -> (56.3658, 4.6871)
  line L119 (56.3658, 4.6871) -> (56.3658, 7.7351)
  line L120 (56.3658, 7.7351) -> (56.9414, 7.7351)
  line L121 (56.9414, 7.7351) -> (58.169, 5.3219)
  line L122 (58.169, 5.3219) -> (58.169, 7.7351)
  line L123 (58.169, 7.7351) -> (58.5469, 7.7351)
  line L124 (58.5469, 7.7351) -> (58.5469, 4.6871)
  spline S188 degree 2 poles (60.4093, 4.9291) (60.3623, 4.8946) (60.2043, 4.7711) (60.1301, 4.734) knots 0 0 0 1 2 2 2
  spline S189 degree 2 poles (60.1301, 4.734) (60.0289, 4.6797) (59.8387, 4.6229) (59.6658, 4.6229) knots 0 0 0 1 2 2 2
  spline S190 degree 2 poles (59.6658, 4.6229) (59.525, 4.6229) (59.2706, 4.7291) (59.1743, 4.8254) knots 0 0 0 1 2 2 2
  spline S191 degree 2 poles (59.1743, 4.8254) (59.0829, 4.9193) (58.9717, 5.1959) (58.9717, 5.349) knots 0 0 0 1 2 2 2
  spline S192 degree 2 poles (58.9717, 5.349) (58.9717, 5.5862) (59.1718, 5.9221) (59.3891, 6.0184) knots 0 0 0 1 2 2 2
  spline S193 degree 2 poles (59.3891, 6.0184) (59.5818, 6.1073) (60.1054, 6.174) (60.4093, 6.1913) knots 0 0 0 1 2 2 2
  line L125 (60.4093, 6.1913) -> (60.4093, 6.2654)
  spline S194 degree 2 poles (60.4093, 6.2654) (60.4093, 6.3988) (60.3278, 6.5643) (60.2537, 6.6112) knots 0 0 0 1 2 2 2
  spline S195 degree 2 poles (60.2537, 6.6112) (60.1796, 6.6581) (59.9671, 6.6878) (59.8535, 6.6878) knots 0 0 0 1 2 2 2
  spline S196 degree 2 poles (59.8535, 6.6878) (59.7201, 6.6878) (59.3595, 6.6087) (59.1792, 6.5322) knots 0 0 0 1 2 2 2
  line L126 (59.1792, 6.5322) -> (59.157, 6.5322)
  line L127 (59.157, 6.5322) -> (59.157, 6.9249)
  spline S197 degree 2 poles (59.157, 6.9249) (59.2632, 6.9546) (59.6608, 7.0287) (59.856, 7.0287) knots 0 0 0 1 2 2 2
  spline S198 degree 2 poles (59.856, 7.0287) (60.0931, 7.0287) (60.4167, 6.9546) (60.5451, 6.8582) knots 0 0 0 1 2 2 2
  spline S199 degree 2 poles (60.5451, 6.8582) (60.6711, 6.7644) (60.7946, 6.4655) (60.7946, 6.2506) knots 0 0 0 1 2 2 2
  line L128 (60.7946, 6.2506) -> (60.7946, 4.6871)
  line L129 (60.7946, 4.6871) -> (60.4093, 4.6871)
  line L130 (60.4093, 4.6871) -> (60.4093, 4.9291)
  line L131 (60.4093, 5.2502) -> (60.4093, 5.885)
  spline S200 degree 2 poles (60.4093, 5.885) (60.2709, 5.8727) (59.8535, 5.8307) (59.7226, 5.7912) knots 0 0 0 1 2 2 2
  spline S201 degree 2 poles (59.7226, 5.7912) (59.5695, 5.7442) (59.3694, 5.5491) (59.3694, 5.3762) knots 0 0 0 1 2 2 2
  spline S202 degree 2 poles (59.3694, 5.3762) (59.3694, 5.1786) (59.5917, 4.9785) (59.8041, 4.9785) knots 0 0 0 1 2 2 2
  spline S203 degree 2 poles (59.8041, 4.9785) (59.9844, 4.9785) (60.2808, 5.1341) (60.4093, 5.2502) knots 0 0 0 1 2 2 2
  line L132 (63.929, 4.6871) -> (63.929, 6.011)
  spline S204 degree 2 poles (63.929, 6.011) (63.929, 6.1691) (63.9043, 6.4383) (63.8648, 6.5124) knots 0 0 0 1 2 2 2
  spline S205 degree 2 poles (63.8648, 6.5124) (63.8253, 6.5939) (63.6746, 6.673) (63.5437, 6.673) knots 0 0 0 1 2 2 2
  spline S206 degree 2 poles (63.5437, 6.673) (63.4252, 6.673) (63.1534, 6.5272) (63.0102, 6.3889) knots 0 0 0 1 2 2 2
  spline S207 degree 2 poles (63.0102, 6.3889) (63.0127, 6.3543) (63.0176, 6.258) (63.0176, 6.1938) knots 0 0 0 1 2 2 2
  line L133 (63.0176, 6.1938) -> (63.0176, 4.6871)
  line L134 (63.0176, 4.6871) -> (62.6323, 4.6871)
  line L135 (62.6323, 4.6871) -> (62.6323, 6.011)
  spline S208 degree 2 poles (62.6323, 6.011) (62.6323, 6.1691) (62.6076, 6.4383) (62.5681, 6.5124) knots 0 0 0 1 2 2 2
  spline S209 degree 2 poles (62.5681, 6.5124) (62.5285, 6.5939) (62.3779, 6.673) (62.247, 6.673) knots 0 0 0 1 2 2 2
  spline S210 degree 2 poles (62.247, 6.673) (62.1235, 6.673) (61.8493, 6.5174) (61.7208, 6.3963) knots 0 0 0 1 2 2 2
  line L136 (61.7208, 6.3963) -> (61.7208, 4.6871)
  line L137 (61.7208, 4.6871) -> (61.3355, 4.6871)
  line L138 (61.3355, 4.6871) -> (61.3355, 6.9743)
  line L139 (61.3355, 6.9743) -> (61.7208, 6.9743)
  line L140 (61.7208, 6.9743) -> (61.7208, 6.7224)
  spline S211 degree 2 poles (61.7208, 6.7224) (61.8715, 6.873) (62.1679, 7.0385) (62.3458, 7.0385) knots 0 0 0 1 2 2 2
  spline S212 degree 2 poles (62.3458, 7.0385) (62.5483, 7.0385) (62.862, 6.8533) (62.9435, 6.6433) knots 0 0 0 1 2 2 2
  spline S213 degree 2 poles (62.9435, 6.6433) (63.1189, 6.8385) (63.4499, 7.0385) (63.6425, 7.0385) knots 0 0 0 1 2 2 2
  spline S214 degree 2 poles (63.6425, 7.0385) (63.7907, 7.0385) (64.0328, 6.9471) (64.1217, 6.8434) knots 0 0 0 1 2 2 2
  spline S215 degree 2 poles (64.1217, 6.8434) (64.2131, 6.7397) (64.3144, 6.4284) (64.3144, 6.1938) knots 0 0 0 1 2 2 2
  line L141 (64.3144, 6.1938) -> (64.3144, 4.6871)
  line L142 (64.3144, 4.6871) -> (63.929, 4.6871)
  spline S216 degree 2 poles (65.8482, 4.6352) (65.2999, 4.6352) (64.6972, 5.2502) (64.6972, 5.8183) knots 0 0 0 1 2 2 2
  spline S217 degree 2 poles (64.6972, 5.8183) (64.6972, 6.3766) (65.2826, 7.0385) (65.7544, 7.0385) knots 0 0 0 1 2 2 2
  spline S218 degree 2 poles (65.7544, 7.0385) (65.9668, 7.0385) (66.2953, 6.915) (66.4163, 6.7841) knots 0 0 0 1 2 2 2
  spline S219 degree 2 poles (66.4163, 6.7841) (66.5398, 6.6532) (66.6708, 6.2753) (66.6708, 6.0011) knots 0 0 0 1 2 2 2
  line L143 (66.6708, 6.0011) -> (66.6708, 5.7912)
  line L144 (66.6708, 5.7912) -> (65.0875, 5.7912)
  spline S220 degree 2 poles (65.0875, 5.7912) (65.0875, 5.3935) (65.4876, 4.9711) (65.8433, 4.9711) knots 0 0 0 1 2 2 2
  spline S221 degree 2 poles (65.8433, 4.9711) (65.9693, 4.9711) (66.2138, 5.0279) (66.3126, 5.0724) knots 0 0 0 1 2 2 2
  spline S222 degree 2 poles (66.3126, 5.0724) (66.4163, 5.1218) (66.5596, 5.2082) (66.6065, 5.2478) knots 0 0 0 1 2 2 2
  line L145 (66.6065, 5.2478) -> (66.6288, 5.2478)
  line L146 (66.6288, 5.2478) -> (66.6288, 4.8279)
  spline S223 degree 2 poles (66.6288, 4.8279) (66.5621, 4.8007) (66.3595, 4.7217) (66.2805, 4.6994) knots 0 0 0 1 2 2 2
  spline S224 degree 2 poles (66.2805, 4.6994) (66.1693, 4.6673) (65.9866, 4.6352) (65.8482, 4.6352) knots 0 0 0 1 2 2 2
  spline S225 degree 2 poles (66.2953, 6.0851) (66.2904, 6.2407) (66.2261, 6.468) (66.1644, 6.5445) knots 0 0 0 1 2 2 2
  spline S226 degree 2 poles (66.1644, 6.5445) (66.0977, 6.631) (65.8878, 6.7224) (65.7321, 6.7224) knots 0 0 0 1 2 2 2
  spline S227 degree 2 poles (65.7321, 6.7224) (65.579, 6.7224) (65.3641, 6.631) (65.2752, 6.5421) knots 0 0 0 1 2 2 2
  spline S228 degree 2 poles (65.2752, 6.5421) (65.1887, 6.4507) (65.0998, 6.2308) (65.0875, 6.0851) knots 0 0 0 1 2 2 2
  line L147 (65.0875, 6.0851) -> (66.2953, 6.0851)
  point P0 (0, 5.7603)
  constraints: 2 other
extrude "Extrusion3" cut sketch "Sketch4" against normal blind 0.254
sketch "Sketch5" plane through (0, 6.6514, 76.2) normal (0.8660254, 0.5, 0) x (0, 0, -1)
  line L0 (67.0697, -2.2328) -> (67.0697, -9.3892)
  line L1 (9.3366, -9.3892) -> (67.0697, -9.3892)
  line L2 (67.0697, -2.2328) -> (9.3366, -2.2328)
  line L3 (9.3366, -2.2328) -> (9.3366, -9.3892)
  line L4 (67.0697, -5.811) -> (76.4063, -5.811) construction
  line L5 (0, -5.7603) -> (9.3366, -5.7603) construction
  constraints: 12 end point, 1 horizontal, 1 midpoint, 1 parallel, 1 perpendicular, 1 point on line, 1 vertical
extrude "Extrusion4" add sketch "Sketch5" along normal blind 0.2286